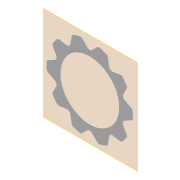
# Autodesk Inventor part: Anglerfish_3inch_tube_rubberring
Saved by Autodesk Inventor 2022 (Build 260153000, 153)
## iProperties
Created: 2022-04-17
Part Number: Anglerfish_3inch_tube_rubberring
Material: Generic
Document SubType Name: Modeling
Designer: Prakash Lab
Density: 1 g/cm^3
Appearance: Default
Author: Prakash Lab
Autodesk Inventor part; units mm, degrees
ref_plane "YZ Plane" through (0, 0, 0) normal (1, 0, 0) x (0, 1, 0)
ref_plane "XZ Plane" through (0, 0, 0) normal (0, 1, 0) x (-1, 0, 0)
ref_plane "XY Plane" through (0, 0, 0) normal (0, 0, 1) x (1, 0, 0)
ref_plane "Work Plane1" through (0, 0, -4) normal (0, 0, 1) x (1, 0, 0)
sketch "Sketch1" plane through (0, 0, -4) normal (0, 0, 1) x (1, 0, 0)
  circle A0 centre (0.1176, -0.1618) radius 38.1 projected
  circle A1 centre (0, 0) radius 43.6 projected
  circle A2 centre (0, 0) radius 55.6 projected
  point P0 (0, 0)
extrude "Extrusion1" add sketch "Sketch1" along normal blind 1 contours A1 | A2
sketch "Sketch2" plane through (0, 0, -3) normal (0, 0, 1) x (1, 0, 0)
  circle A0 centre (47.1724, 15.3272) radius 2 projected
  circle A1 centre (47.1724, 15.3272) radius 4.4912
  line L0 (45.1335, 11.3256) -> (55.2569, 6.1675)
  circle A2 centre (0, 0) radius 55.6 projected
  line L1 (43.1708, 17.3662) -> (48.3289, 27.4896)
  line L2 (47.1724, 15.3272) -> (52.8787, 17.1813)
  point P0 (0, 0)
  dimension "d2" = 45
  dimension "d3" = 45
  constraints: 6 end point, 5 point on circle, 2 tangent, 1 centre point, 1 line through centre
  measures "d2" angle of L2 L1
  measures "d3" angle of L2 L0
extrude "Extrusion2" cut sketch "Sketch2" against normal blind 1 contours A0 | A1 | L1 A2 L2 A1 | A1 L2 A2 L0
fillet "Fillet1" radius 4 2 edges at (48.3289, 27.4896, -3.5) (55.2569, 6.1675, -3.5)
pattern_circular "Circular Pattern1" count 10 over 360 about axis through (0, 0, -4) along (0, 0, 1) of "Extrusion2", "Fillet1"
equation "\"d3\" = d2"
body "Solid1"
